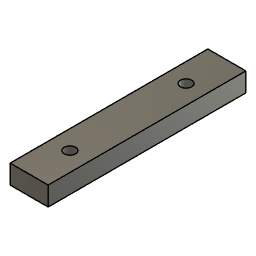
LED_NEON_COLON (Autodesk Fusion 360 design; units mm, degrees)
Autodesk Fusion 360 part; units mm, degrees
note: some values were not read from the file. Set by a fixed rule: the direction of a hole.
sketch "Sketch1" plane through (0, 0, 0) normal (0, 1, 0) x (1, 0, 0)
  line L0 (-9, 46.8) -> (9, 46.8)
  line L1 (9, 46.8) -> (9, -46.8)
  line L2 (9, -46.8) -> (-9, -46.8)
  line L3 (-9, -46.8) -> (-9, 46.8)
  line L4 (0, 46.8) -> (0, -46.8) construction
  line L5 (0, 27.5) -> (0, -27.5) construction
  point P0 (0, 27.5)
  point P1 (0, -27.5)
  dimension "d1" = 18
  dimension "d2" = 93.6
  dimension "d3" = 55
  constraint horizontal L0
  constraint vertical L1
  constraint horizontal L2
  constraint vertical L3
  constraint midpoint L0 L4.start
  constraint midpoint L2 L4.end
  constraint midpoint origin L4
  constraint coincident L4 P0
  constraint coincident L4 P1
  constraint parallel L4 L5
  constraint midpoint origin L5
  constraint coincident P0 L5.start
  constraint coincident P1 L5.end
  measures "d1" distance of L1.end L2.end
  measures "d2" distance of L0.end L1.end
  measures "d3" distance of P0 P1
sketch "Sketch2" plane through (0, 0, 0) normal (0, 0, 1) x (1, 0, 0)
  line L0 (9, 0) -> (-9, 0)
  line L1 (9, 0) -> (9, 9)
  line L2 (9, 9) -> (-9, 9)
  line L3 (-9, 9) -> (-9, 0)
  point P0 (9, 0)
  dimension "d4" = 9
  constraint coincident P0 L0.start
  constraint horizontal L0
  constraint midpoint L0 origin
  constraint perpendicular L0 L1
  constraint perpendicular L1 L2
  constraint vertical L3
  measures "d4" distance of P0 L1.end
extrude "Extrude1" add sketch "Sketch1" along normal up to surface (9 mm away)
hole "Hole1" at (0, 0, 27.5) at (0, 0, -27.5) direction (0, 1, 0) diameter 5.4 end up to surface (9 mm away)
